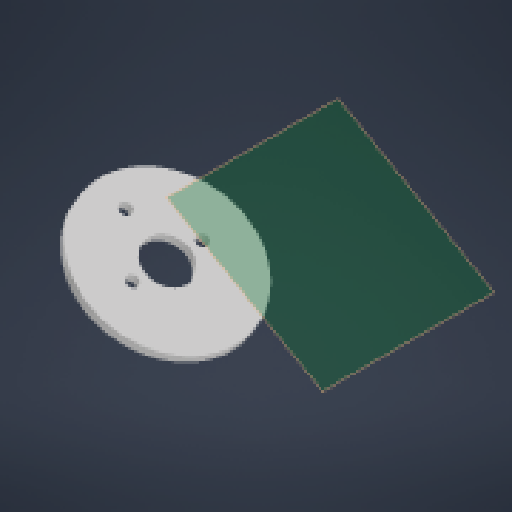
# Autodesk Inventor part: Head3MotorsSustain
Saved by Autodesk Inventor 2026 (Build 300175050, 175E)
## iProperties
Created: 2025-07-17
Part Number: Head3MotorsSustain
Material: Generic
Document SubType Name: Modeling
Designer: RubenPC
Density: 1 g/cm^3
Appearance: Default
Author: RubenPC
Autodesk Inventor part; units mm, degrees
ref_plane "YZ Plane" through (0, 0, 0) normal (1, 0, 0) x (0, 1, 0)
ref_plane "XZ Plane" through (0, 0, 0) normal (0, 1, 0) x (-1, 0, 0)
ref_plane "XY Plane" through (0, 0, 0) normal (0, 0, 1) x (1, 0, 0)
ref_plane "Work Plane2" through (44.6963, -1.706, 47.3296) normal (-0.5, -0.8660254, 0) x (0.8660254, -0.5, 0)
sketch "Sketch2" plane through (44.6963, -1.706, 47.3296) normal (-0.5, -0.8660254, 0) x (0.8660254, -0.5, 0)
  circle A0 centre (0, 0) radius 13.35 projected
  circle A1 centre (0, -8) radius 1.3 projected
  circle A2 centre (0, 8) radius 1.3 projected
  circle A3 centre (-11, 0) radius 1.3 projected
  circle A4 centre (0, 0) radius 5 projected
  circle A5 centre (0, 0) radius 17.9909
  point P0 (-39.5612, -47.3296)
  constraints: 1 centre point, 1 coincident
ref_plane "Work Plane3" through (-49.8037, -1.706, 47.3296) normal (0.5, -0.8660254, 0) x (0.8660254, 0.5, 0)
sketch "Sketch3" plane through (-49.8037, -1.706, 47.3296) normal (0.5, -0.8660254, 0) x (0.8660254, 0.5, 0)
  circle A0 centre (0, 0) radius 13.35 projected
  circle A1 centre (0, -8) radius 1.3 projected
  circle A2 centre (0, 8) radius 1.3 projected
  circle A3 centre (-11, 0) radius 1.3 projected
  circle A4 centre (0, 0) radius 5 projected
  circle A5 centre (0, 0) radius 18.419
  point P0 (43.9843, -47.3296)
  constraints: 1 centre point, 1 coincident
ref_plane "Work Plane4" through (-9.0537, 68.191, 47.3296) normal (1, 0, 0) x (0, 1, 0)
sketch "Sketch4" plane through (-9.0537, 68.191, 47.3296) normal (1, 0, 0) x (0, 1, 0)
  circle A0 centre (0, 0) radius 13.35 projected
  circle A1 centre (0, -8) radius 1.3 projected
  circle A2 centre (0, 8) radius 1.3 projected
  circle A3 centre (-11, 0) radius 1.3 projected
  circle A4 centre (0, 0) radius 5 projected
  circle A5 centre (0, 0) radius 18.4138
  point P0 (-68.191, -47.3296)
  constraints: 1 centre point, 1 coincident
extrude "Extrusion2" add sketch "Sketch2" along normal blind 2 contours A0 | A1 | A2 | A3 | A4 | A5
extrude "Extrusion3" add sketch "Sketch3" along normal blind 2 contours A0 | A5
ref_plane "Work Plane5" through (-2.5537, 18.0682, 27.3296) normal (0, 0, 1) x (1, 0, 0)
sketch "Sketch5" plane through (-2.5537, 18.0682, 27.3296) normal (0, 0, 1) x (1, 0, 0)
  spline S0 degree 3 poles (0, 29.8062) (0.9457, 29.8062) (1.8876, 29.7588) (2.8246, 29.6646) (3.7616, 29.5705) (4.6943, 29.4294) (5.6219, 29.241) (6.0858, 29.1467) (6.5493, 29.0403) (7.0101, 28.9222) (7.471, 28.804) (7.9259, 28.675) (8.3761, 28.5351) (8.8263, 28.3951) (9.2714, 28.2444) (9.7115, 28.0831) (10.1517, 27.9218) (10.5869, 27.7498) (11.0172, 27.5673) (11.8778, 27.2024) (12.7194, 26.7951) (13.5409, 26.346) (13.9517, 26.1215) (14.3579, 25.8862) (14.7594, 25.64) (15.1609, 25.3939) (15.555, 25.1386) (15.9409, 24.8749) (16.7126, 24.3474) (17.4541, 23.7852) (18.1655, 23.1894) (18.8769, 22.5936) (19.5586, 21.9639) (20.2104, 21.3008) (20.5363, 20.9692) (20.855, 20.6289) (21.1659, 20.2804) (21.4767, 19.9319) (21.781, 19.5738) (22.0756, 19.2093) (22.3702, 18.8449) (22.6547, 18.4749) (22.9298, 18.099) (23.2048, 17.723) (23.4702, 17.3414) (23.7261, 16.954) (24.2378, 16.1793) (24.7115, 15.3819) (25.1472, 14.5621) (25.5829, 13.7422) (25.9807, 12.8996) (26.3394, 12.0345) (26.5188, 11.602) (26.6886, 11.1628) (26.848, 10.7195) (27.0073, 10.2761) (27.1551, 9.831) (27.2921, 9.3834) (27.4291, 8.9358) (27.555, 8.486) (27.67, 8.034) (27.785, 7.5821) (27.8891, 7.1279) (27.9823, 6.6716) (28.1687, 5.7589) (28.3117, 4.8377) (28.4107, 3.9079) (28.5096, 2.9781) (28.5646, 2.0404) (28.5737, 1.0927) (28.5828, 0.145) (28.5457, -0.7973) (28.4639, -1.7318) (28.3822, -2.6663) (28.2557, -3.5939) (28.0846, -4.5144) (27.999, -4.9746) (27.9023, -5.4331) (27.7944, -5.8898) (27.6864, -6.3464) (27.5672, -6.8013) (27.4365, -7.2544) (27.3059, -7.7074) (27.1639, -8.1584) (27.01, -8.6079) (26.8562, -9.0575) (26.691, -9.5039) (26.5158, -9.9436) (26.1656, -10.823) (25.7744, -11.6801) (25.3432, -12.5148) (24.9119, -13.3495) (24.4406, -14.1621) (23.9288, -14.9522) (23.673, -15.3472) (23.407, -15.7366) (23.1307, -16.1204) (22.8545, -16.5041) (22.5681, -16.8819) (22.2709, -17.2543) (21.9738, -17.6267) (21.6669, -17.9922) (21.3529, -18.3477) (21.039, -18.7033) (20.717, -19.0502) (20.3875, -19.3881) (19.7285, -20.0639) (19.0385, -20.7047) (18.318, -21.3106) (17.9577, -21.6135) (17.5898, -21.9077) (17.2142, -22.1931) (16.8386, -22.4785) (16.4553, -22.755) (16.0641, -23.0227) (15.673, -23.2903) (15.2742, -23.5488) (14.867, -23.7985) (14.4598, -24.0482) (14.0471, -24.2872) (13.6306, -24.5146) (12.7976, -24.9695) (11.9466, -25.3805) (11.0786, -25.7478) (10.2106, -26.1152) (9.3253, -26.4391) (8.4228, -26.7192) (7.5202, -26.9993) (6.5996, -27.2357) (5.6624, -27.4263) (4.7252, -27.6169) (3.7842, -27.7592) (2.8377, -27.8543) (1.8911, -27.9493) (0.9396, -27.9969) (-0.0167, -27.9963) (-0.9731, -27.9958) (-1.9211, -27.9471) (-2.8612, -27.8519) (-3.8013, -27.7567) (-4.7335, -27.6151) (-5.6578, -27.4273) (-6.5821, -27.2394) (-7.4985, -27.0054) (-8.4067, -26.7242) (-8.8609, -26.5836) (-9.3141, -26.4306) (-9.7622, -26.2667) (-10.2104, -26.1028) (-10.6522, -25.9284) (-11.0885, -25.7436) (-11.5248, -25.5588) (-11.9553, -25.3636) (-12.3801, -25.1581) (-12.8049, -24.9526) (-13.224, -24.7368) (-13.6374, -24.5109) (-14.0509, -24.2849) (-14.4586, -24.0488) (-14.8607, -23.8024) (-15.2628, -23.556) (-15.6591, -23.2994) (-16.0498, -23.0325) (-16.4404, -22.7656) (-16.8254, -22.4882) (-17.2044, -22.2006) (-17.5833, -21.9129) (-17.9574, -21.6139) (-18.3212, -21.3079) (-18.685, -21.0019) (-19.0402, -20.6876) (-19.3864, -20.3657) (-19.7325, -20.0438) (-20.07, -19.7141) (-20.3987, -19.3767) (-21.0561, -18.7018) (-21.6788, -17.996) (-22.2668, -17.2595) (-22.5608, -16.8913) (-22.8461, -16.5153) (-23.1226, -16.1316) (-23.3992, -15.7479) (-23.6668, -15.3566) (-23.9257, -14.9569) (-24.1847, -14.5573) (-24.4339, -14.1509) (-24.6715, -13.741) (-24.9091, -13.3311) (-25.136, -12.9164) (-25.3521, -12.4976) (-25.7841, -11.6599) (-26.1735, -10.8044) (-26.5206, -9.9317) (-26.8676, -9.0591) (-27.1725, -8.1686) (-27.4344, -7.2617) (-27.5654, -6.8082) (-27.6856, -6.35) (-27.7949, -5.8873) (-27.9043, -5.4247) (-28.0019, -4.961) (-28.0878, -4.4971) (-28.2596, -3.5694) (-28.3854, -2.6385) (-28.4662, -1.7056) (-28.547, -0.7727) (-28.5828, 0.1625) (-28.5736, 1.0999) (-28.5644, 2.0373) (-28.51, 2.9775) (-28.4095, 3.9186) (-28.309, 4.8598) (-28.164, 5.7871) (-27.976, 6.7023) (-27.788, 7.6175) (-27.5572, 8.5202) (-27.2838, 9.4104) (-27.0105, 10.3005) (-26.6946, 11.1784) (-26.336, 12.0428) (-26.1567, 12.475) (-25.9663, 12.9045) (-25.7652, 13.3301) (-25.5641, 13.7557) (-25.3537, 14.1745) (-25.1342, 14.5866) (-24.6951, 15.4107) (-24.219, 16.2097) (-23.7072, 16.9826) (-23.1954, 17.7554) (-22.6476, 18.5027) (-22.0637, 19.2241) (-21.7717, 19.5847) (-21.4706, 19.9389) (-21.1604, 20.2866) (-20.8501, 20.6342) (-20.5309, 20.975) (-20.2018, 21.3096) (-19.8728, 21.6441) (-19.5361, 21.97) (-19.1931, 22.2862) (-18.8502, 22.6024) (-18.5005, 22.9094) (-18.1443, 23.2071) (-17.4318, 23.8027) (-16.6929, 24.3616) (-15.9275, 24.884) (-15.5447, 25.1452) (-15.1554, 25.3973) (-14.7593, 25.6401) (-14.3631, 25.883) (-13.9603, 26.1166) (-13.5505, 26.3408) (-13.1407, 26.565) (-12.724, 26.7799) (-12.3001, 26.9851) (-11.8762, 27.1904) (-11.4449, 27.3861) (-11.0113, 27.5698) (-10.1441, 27.9373) (-9.2641, 28.2593) (-8.3708, 28.5367) (-7.4774, 28.8142) (-6.571, 29.0471) (-5.651, 29.235) (-5.191, 29.329) (-4.7277, 29.4117) (-4.2609, 29.483) (-3.794, 29.5542) (-3.3237, 29.614) (-2.8499, 29.6621) (-2.3761, 29.7101) (-1.8977, 29.7464) (-1.4226, 29.7704) (-0.9475, 29.7943) (-0.4728, 29.8062) (0, 29.8062) knots -1 -1 -1 -1 -0.984375 -0.984375 -0.984375 -0.96875 -0.96875 -0.96875 -0.960938 -0.960938 -0.960938 -0.953125 -0.953125 -0.953125 -0.945312 -0.945312 -0.945312 -0.9375 -0.9375 -0.9375 -0.921875 -0.921875 -0.921875 -0.914062 -0.914062 -0.914062 -0.90625 -0.90625 -0.90625 -0.890625 -0.890625 -0.890625 -0.875 -0.875 -0.875 -0.867188 -0.867188 -0.867188 -0.859375 -0.859375 -0.859375 -0.851562 -0.851562 -0.851562 -0.84375 -0.84375 -0.84375 -0.828125 -0.828125 -0.828125 -0.8125 -0.8125 -0.8125 -0.804688 -0.804688 -0.804688 -0.796875 -0.796875 -0.796875 -0.789062 -0.789062 -0.789062 -0.78125 -0.78125 -0.78125 -0.765625 -0.765625 -0.765625 -0.75 -0.75 -0.75 -0.734375 -0.734375 -0.734375 -0.71875 -0.71875 -0.71875 -0.710938 -0.710938 -0.710938 -0.703125 -0.703125 -0.703125 -0.695312 -0.695312 -0.695312 -0.6875 -0.6875 -0.6875 -0.671875 -0.671875 -0.671875 -0.65625 -0.65625 -0.65625 -0.648438 -0.648438 -0.648438 -0.640625 -0.640625 -0.640625 -0.632812 -0.632812 -0.632812 -0.625 -0.625 -0.625 -0.609375 -0.609375 -0.609375 -0.601562 -0.601562 -0.601562 -0.59375 -0.59375 -0.59375 -0.585938 -0.585938 -0.585938 -0.578125 -0.578125 -0.578125 -0.5625 -0.5625 -0.5625 -0.546875 -0.546875 -0.546875 -0.53125 -0.53125 -0.53125 -0.515625 -0.515625 -0.515625 -0.5 -0.5 -0.5 -0.484375 -0.484375 -0.484375 -0.46875 -0.46875 -0.46875 -0.453125 -0.453125 -0.453125 -0.445312 -0.445312 -0.445312 -0.4375 -0.4375 -0.4375 -0.429688 -0.429688 -0.429688 -0.421875 -0.421875 -0.421875 -0.414062 -0.414062 -0.414062 -0.40625 -0.40625 -0.40625 -0.398438 -0.398438 -0.398438 -0.390625 -0.390625 -0.390625 -0.382812 -0.382812 -0.382812 -0.375 -0.375 -0.375 -0.359375 -0.359375 -0.359375 -0.351563 -0.351563 -0.351563 -0.34375 -0.34375 -0.34375 -0.335938 -0.335938 -0.335938 -0.328125 -0.328125 -0.328125 -0.3125 -0.3125 -0.3125 -0.296875 -0.296875 -0.296875 -0.289063 -0.289063 -0.289063 -0.28125 -0.28125 -0.28125 -0.265625 -0.265625 -0.265625 -0.25 -0.25 -0.25 -0.234375 -0.234375 -0.234375 -0.21875 -0.21875 -0.21875 -0.203125 -0.203125 -0.203125 -0.1875 -0.1875 -0.1875 -0.179688 -0.179688 -0.179688 -0.171875 -0.171875 -0.171875 -0.15625 -0.15625 -0.15625 -0.140625 -0.140625 -0.140625 -0.132812 -0.132812 -0.132812 -0.125 -0.125 -0.125 -0.117187 -0.117187 -0.117187 -0.109375 -0.109375 -0.109375 -0.09375 -0.09375 -0.09375 -0.085937 -0.085937 -0.085937 -0.078125 -0.078125 -0.078125 -0.070313 -0.070313 -0.070313 -0.0625 -0.0625 -0.0625 -0.046875 -0.046875 -0.046875 -0.03125 -0.03125 -0.03125 -0.023438 -0.023438 -0.023438 -0.015625 -0.015625 -0.015625 -0.007813 -0.007813 -0.007813 0 0 0 0 projected
  circle A0 centre (0, 0) radius 24.13 projected
  point P0 (2.5537, -18.0682)
  point P1 (0, 29.8062)
extrude "Extrusion5" add sketch "Sketch4" along normal blind 2 contours A0 | A5
body "Solid2"
